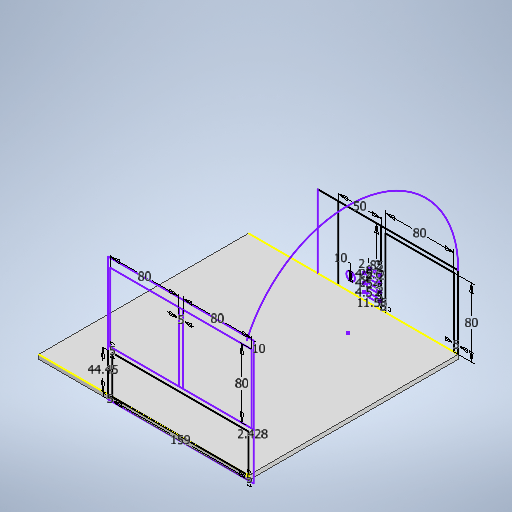
# Autodesk Inventor part: matx-arc-case
Saved by Autodesk Inventor 2025 (Build 290162000, 162)
## iProperties
Created: 2024-07-16
Part Number: matx-arc-case
Material: Generic
Document SubType Name: Modeling
Designer: admin
Density: 1 g/cm^3
Appearance: Default
Author: admin
Autodesk Inventor part; units mm, degrees
ref_plane "YZ Plane" through (0, 0, 0) normal (1, 0, 0) x (0, 1, 0)
ref_plane "XZ Plane" through (0, 0, 0) normal (0, 1, 0) x (-1, 0, 0)
ref_plane "XY Plane" through (0, 0, 0) normal (0, 0, 1) x (1, 0, 0)
sketch "Sketch1" plane through (0, 0, 0) normal (0, 1, 0) x (-1, 0, 0)
  line L0 (0, 0) -> (245, 0)
  line L1 (245, 0) -> (245, -245)
  line L2 (245, -245) -> (0, -245)
  line L3 (0, -245) -> (0, 0)
  dimension "d0" = 245
  dimension "d1" = 245
  constraints: 8 end point, 3 perpendicular, 1 horizontal
  measures "d0" distance of L0.start L0.end
  measures "d1" distance of L0.end L1.end
sketch "Sketch2" plane through (0, 0, 0) normal (0, 0, 1) x (1, 0, 0)
  line L0 (0, 0) -> (-159, 0)
  line L1 (-159, 0) -> (-159, 44.45)
  line L2 (-159, 44.45) -> (0, 44.45)
  line L3 (0, 44.45) -> (0, 0)
  line L4 (-159, 0) -> (-164, 0)
  line L5 (-164, 0) -> (-164, 44.45)
  line L6 (-164, 44.45) -> (-164, 49.45)
  line L7 (-161.4275, 49.45) -> (3.5725, 49.45)
  line L8 (6, 49.45) -> (6, 0)
  line L9 (6, 0) -> (6, -5)
  line L10 (6, -5) -> (-164, -5)
  line L11 (-164, -5) -> (-164, 0)
  line L12 (3.5725, 49.45) -> (3.5725, 129.45)
  line L13 (3.5725, 129.45) -> (-76.4275, 129.45)
  line L14 (-76.4275, 129.45) -> (-76.4275, 49.45)
  line L15 (-76.4275, 129.45) -> (-81.4275, 129.45)
  line L16 (-81.4275, 129.45) -> (-161.4275, 129.45)
  line L17 (-161.4275, 129.45) -> (-161.4275, 49.45)
  line L18 (-164, 49.45) -> (-161.4275, 49.45)
  line L19 (6, 49.45) -> (3.5725, 49.45)
  line L20 (-81.4275, 129.45) -> (-81.4275, 49.45)
  line L21 (-164, 49.45) -> (-164, 129.45)
  line L22 (6, 49.45) -> (6, 129.45)
  line L23 (6, 129.45) -> (6, 139.45)
  line L24 (6, 139.45) -> (-161.4275, 139.45)
  line L25 (-161.4275, 139.45) -> (-164, 139.45)
  line L26 (-164, 139.45) -> (-164, 128.7782)
  dimension "d2" = 159
  dimension "d3" = 44.45
  dimension "d14" = 5
  dimension "d15" = 5
  dimension "d16" = 2.4275
  dimension "d17" = 5
  dimension "d18" = 80
  dimension "d19" = 80
  dimension "d20" = 5
  dimension "d21" = 80
  dimension "d22" = 10
  constraints: 54 end point, 13 perpendicular, 11 point on line, 2 collinear, 1 horizontal, 1 parallel, 1 vertical
  measures "d2" distance of L0.start L0.end
  measures "d3" distance of L0.end L1.end
  measures "d14" distance of L0.end L4.end
  measures "d15" distance of L6.end L5.end
  measures "d16" distance of L7.end L8.start
  measures "d17" distance of L8.end L9.end
  measures "d18" distance of L7.end L12.end
  measures "d19" distance of L12.end L13.end
  measures "d20" distance of L13.end L15.end
  measures "d21" distance of L15.end L16.end
  measures "d22" distance of L22.end L23.end
extrude "Extrusion1" add sketch "Sketch1" against normal blind 5
sketch "Sketch3" plane through (0, 0, 0) normal (0, 0, 1) x (1, 0, 0)
  line L0 (0, 0) -> (-245, 0) projected
sketch "Sketch4" plane through (0, 0, -245) normal (0, 0, -1) x (-1, 0, 0)
  line L0 (0, 0) -> (245, 0) projected
  line L1 (0, 0) -> (5, 0)
  line L2 (5, 0) -> (5, 80)
  line L3 (5, 80) -> (85, 80)
  line L4 (85, 80) -> (85, 0)
  line L5 (85, 0) -> (90, 0)
  line L6 (90, 0) -> (90, 85)
  line L7 (90, 85) -> (0, 85)
  line L8 (0, 85) -> (0, 0)
  line L9 (90, 85) -> (140, 85)
  line L10 (140, 85) -> (140, 0)
  line L11 (140, 85) -> (164.1969, 85)
  line L12 (164.1969, 85) -> (164.1969, 0)
  line L13 (95, 5.5531) -> (106.55, 5.5531)
  line L14 (106.55, 5.5531) -> (106.55, 10.0531)
  line L15 (106.55, 10.0531) -> (95, 10.0531)
  line L16 (95, 10.0531) -> (95, 5.5531)
  line L17 (95, 15.0531) -> (106.55, 15.0531)
  line L18 (106.55, 15.0531) -> (106.55, 19.5531)
  line L19 (106.55, 19.5531) -> (95, 19.5531)
  line L20 (95, 19.5531) -> (95, 15.0531)
  line L21 (95, 24.5531) -> (106.55, 24.5531)
  line L22 (106.55, 24.5531) -> (106.55, 29.0531)
  line L23 (106.55, 29.0531) -> (95, 29.0531)
  line L24 (95, 29.0531) -> (95, 24.5531)
  line L25 (93.2932, 33.5295) -> (101.6932, 33.5295)
  line L26 (101.6932, 33.5295) -> (101.6932, 36.1295)
  line L27 (101.6932, 36.1295) -> (93.2932, 36.1295)
  line L28 (93.2932, 36.1295) -> (93.2932, 33.5295)
  circle A0 centre (110.1215, 7.8031) radius 1
  circle A1 centre (110.1215, 17.3031) radius 1
  circle A2 centre (110.1215, 26.8031) radius 1
  circle A3 centre (103.2902, 34.8295) radius 1
  circle A4 centre (91.7455, 7.8031) radius 1
  circle A5 centre (91.7455, 17.3031) radius 1
  circle A6 centre (91.7455, 26.8031) radius 1
  circle A7 centre (91.5305, 34.8295) radius 1
  circle A8 centre (125.6793, 16.3031) radius 5
  dimension "d25" = 5
  dimension "d26" = 80
  dimension "d27" = 80
  dimension "d28" = 5
  dimension "d29" = 85
  dimension "d30" = 50
  dimension "d32" = 11.55
  dimension "d33" = 4.5
  dimension "d34" = 5
  dimension "d35" = 4.5
  dimension "d36" = 5
  dimension "d37" = 4.5
  dimension "d38" = 8.4
  dimension "d39" = 2.6
  dimension "d40" = 2
  dimension "d41" = 2
  dimension "d42" = 2
  dimension "d43" = 2
  dimension "d44" = 2
  dimension "d45" = 2
  dimension "d46" = 2
  dimension "d47" = 2
  dimension "d48" = 10
  constraints: 56 end point, 14 perpendicular, 11 point on line, 9 centre point, 3 vertical, 2 horizontal, 1 parallel
  measures "d25" distance of L0.start L1.end
  measures "d26" distance of L1.end L2.end
  measures "d27" distance of L2.end L3.end
  measures "d28" distance of L4.end L5.end
  measures "d29" distance of L5.end L6.end
  measures "d30" distance of L6.end L9.end
  measures "d32" distance of L13.start L13.end
  measures "d33" distance of L13.end L14.end
  measures "d34" distance of L15.end L17.start
  measures "d35" distance of L17.end L18.end
  measures "d36" distance of L19.end L21.start
  measures "d37" distance of L21.end L22.end
  measures "d38" distance of L25.start L25.end
  measures "d39" distance of L25.end L26.end
  measures "d40" diameter of A0
  measures "d41" diameter of A1
  measures "d42" diameter of A2
  measures "d43" diameter of A3
  measures "d44" diameter of A4
  measures "d45" diameter of A5
  measures "d46" diameter of A6
  measures "d47" diameter of A7
  measures "d48" diameter of A8
sketch "Sketch5" plane through (0, 0, 0) normal (0, 1, 0) x (1, 0, 0)
  point P0 (0, 0)
sketch "Sketch6" plane through (0, 0, 0) normal (1, 0, 0) x (0, 0, -1)
  arc A0 (245, 85) -> (-2.0068, 137.6052) centre (116.0975, 85.9509) ccw
  point P0 (0, 0)
  constraints: 2 point on circle, 1 centre point
body "Solid1"
